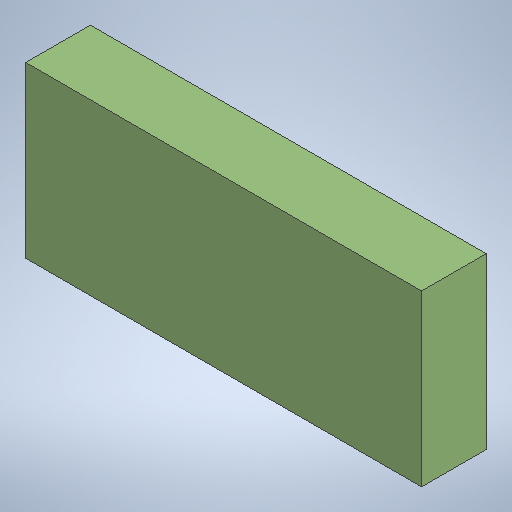
# Autodesk Inventor part: LiFe Battery Blockout v0.1
Saved by Autodesk Inventor 2025 (Build 290162000, 162)
## iProperties
Created: 2024-06-07
Part Number: LiFe Battery Blockout v0.1
Material: Generic
Document SubType Name: Modeling
Designer: sgols
Density: 1 g/cm^3
Appearance: Default
Author: sgols
Autodesk Inventor part; units mm, degrees
ref_plane "YZ Plane" through (0, 0, 0) normal (1, 0, 0) x (0, 1, 0)
ref_plane "XZ Plane" through (0, 0, 0) normal (0, 1, 0) x (-1, 0, 0)
ref_plane "XY Plane" through (0, 0, 0) normal (0, 0, 1) x (1, 0, 0)
sketch "Sketch1" plane through (0, 0, 0) normal (0, 0, 1) x (1, 0, 0)
  line L0 (-49, -21) -> (49, -21)
  line L1 (49, -21) -> (49, 21)
  line L2 (49, 21) -> (-49, 21)
  line L3 (-49, 21) -> (-49, -21)
  line L4 (-49, -21) -> (49, 21) construction
  line L5 (49, -21) -> (-49, 21) construction
  point P0 (0, 0)
  dimension "d0" = 98
  dimension "d1" = 42
  constraints: 12 end point, 2 midpoint, 2 parallel, 1 horizontal, 1 perpendicular
  measures "d0" distance of L0.start L0.end
  measures "d1" distance of L0.end L1.end
extrude "Extrusion1" add sketch "Sketch1" along normal mid plane 16
body "Solid1"
